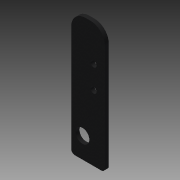
# Autodesk Inventor part: z_screw_bottom_mount
Saved by Autodesk Inventor 2013 SP2 (Build 170200200, 200)
## iProperties
Created: 2013-05-31
Part Number: z_screw_bottom_mount
Material: Steel, Mild
Document SubType Name: Modeling
Designer: Edward
Density: 7.86 g/cm^3
Vendor: custom
Mass: 81.6562 g
Surface Area: 72.357 cm^2
Volume: 10.3888 cm^3
Stock Number: SM_Z2
Description: z-axis bearing mount (bottom)
Author: Edward
Autodesk Inventor part; units mm, degrees
ref_plane "YZ Plane" through (0, 0, 0) normal (1, 0, 0) x (0, 1, 0)
ref_plane "XZ Plane" through (0, 0, 0) normal (0, 1, 0) x (-1, 0, 0)
ref_plane "XY Plane" through (0, 0, 0) normal (0, 0, 1) x (1, 0, 0)
sketch "Sketch1" plane through (0, 0, 0) normal (0, 0, 1) x (1, 0, 0)
  line L0 (-19.4806, -69.0981) -> (-16.0643, -69.0981) projected
  line L1 (-16.0643, 40.9019) -> (-19.4806, 40.9019) projected
  circle A0 centre (0.3057, -10.8501) radius 2.65 projected
  circle A1 centre (0.3057, 9.1499) radius 2.65 projected
  line L2 (-19.4806, -64.0981) -> (-19.4806, 35.9019) projected
  line L3 (60.4357, -17.8501) -> (60.4357, 16.1499) projected
  arc A2 (32.4357, 9.8999) -> (32.4357, -11.6001) centre (32.4357, -0.8501) ccw projected
  circle A3 centre (-9.5643, -50.8501) radius 6.125 projected
  line L4 (10.3057, 75.9749) -> (10.3057, -77.6751) projected
  line L5 (-19.4806, -69.0981) -> (10.3057, -69.0981)
  line L6 (10.3057, -69.0981) -> (10.3057, 40.9019)
  line L7 (10.3057, 40.9019) -> (-19.4806, 40.9019)
  line L8 (-19.4806, 40.9019) -> (-19.4806, -69.0981)
  point P0 (0, 0)
  constraints: 8 end point, 2 parallel, 1 horizontal, 1 perpendicular, 1 point on line
extrude "Extrusion1" add sketch "Sketch1" along normal blind 3.4163
fillet "Fillet1" radius 3.175 2 edges at (10.3057, -69.0981, 1.7082) (-19.4806, -69.0981, 1.7082)
fillet "Fillet2" radius 12.7 2 edges at (-19.4806, 40.9019, 1.7082) (10.3057, 40.9019, 1.7082)
body "Solid1"
